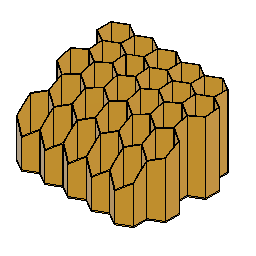
HEXAGON-10 (Autodesk Fusion 360 design; units mm, degrees)
Autodesk Fusion 360 part; units mm, degrees
note: some values were not read from the file. Set by a fixed rule: which sketch regions a step uses.
sketch "Sketch1" plane through (0, 0, 0) normal (0, 1, 0) x (1, 0, 0)
  line L0 (16, 9.2376) -> (0, 18.4752)
  line L1 (0, 18.4752) -> (-16, 9.2376)
  line L2 (-16, -9.2376) -> (0, -18.4752)
  line L3 (0, -18.4752) -> (16, -9.2376)
  line L4 (16, -9.2376) -> (16, 9.2376)
  line L5 (32, -18.4752) -> (48, -9.2376)
  line L6 (48, 9.2376) -> (32, 18.4752)
  line L7 (16, 9.2376) -> (16, -9.2376)
  line L8 (48, -9.2376) -> (48, 9.2376)
  line L9 (32, 18.4752) -> (16, 9.2376)
  line L10 (16, -9.2376) -> (32, -18.4752)
  line L11 (64, -18.4752) -> (80, -9.2376)
  line L12 (80, 9.2376) -> (64, 18.4752)
  line L13 (48, 9.2376) -> (48, -9.2376)
  line L14 (80, -9.2376) -> (80, 9.2376)
  line L15 (64, 18.4752) -> (48, 9.2376)
  line L16 (48, -9.2376) -> (64, -18.4752)
  line L17 (96, -18.4752) -> (112, -9.2376)
  line L18 (112, 9.2376) -> (96, 18.4752)
  line L19 (80, 9.2376) -> (80, -9.2376)
  line L20 (112, -9.2376) -> (112, 9.2376)
  line L21 (96, 18.4752) -> (80, 9.2376)
  line L22 (80, -9.2376) -> (96, -18.4752)
  line L23 (128, -18.4752) -> (144, -9.2376)
  line L24 (144, 9.2376) -> (128, 18.4752)
  line L25 (112, 9.2376) -> (112, -9.2376)
  line L26 (144, -8.7757) -> (144, 9.2376)
  line L27 (128, 18.4752) -> (112, 9.2376)
  line L28 (112, -9.2376) -> (128, -18.4752)
  line L29 (-16, 9.2376) -> (-16, -9.2376)
  line L30 (16, -9.2376) -> (0, -18.4752)
  line L31 (0, -18.4752) -> (0, -36.9504)
  line L32 (0, -36.9504) -> (16, -46.188)
  line L33 (16, -46.188) -> (32, -36.9504)
  line L34 (32, -36.9504) -> (32, -18.4752)
  line L35 (32, -18.4752) -> (16, -9.2376)
  line L36 (32, -18.4752) -> (32, -36.9504)
  line L37 (32, -36.9504) -> (48, -46.188)
  line L38 (48, -46.188) -> (64, -36.9504)
  line L39 (64, -36.9504) -> (64, -18.4752)
  line L40 (64, -18.4752) -> (48, -9.2376)
  line L41 (48, -9.2376) -> (32, -18.4752)
  line L42 (64, -18.4752) -> (64, -36.9504)
  line L43 (64, -36.9504) -> (80, -46.188)
  line L44 (80, -46.188) -> (96, -36.9504)
  line L45 (96, -36.9504) -> (96, -18.4752)
  line L46 (96, -18.4752) -> (80, -9.2376)
  line L47 (80, -9.2376) -> (64, -18.4752)
  line L48 (112, -9.2376) -> (96, -18.4752)
  line L49 (96, -18.4752) -> (96, -36.9504)
  line L50 (96, -36.9504) -> (112, -46.188)
  line L51 (112, -46.188) -> (128, -36.9504)
  line L52 (128, -36.9504) -> (128, -18.4752)
  line L53 (128, -18.4752) -> (112, -9.2376)
  line L54 (128, -18.4752) -> (128, -36.9504)
  line L55 (128, -36.9504) -> (144, -46.188)
  line L56 (144, -46.188) -> (160, -36.9504)
  line L57 (160, -36.9504) -> (160, -18.4752)
  line L58 (160, -18.4752) -> (144, -9.2376)
  line L59 (144, -9.2376) -> (128, -18.4752)
  line L60 (0, -36.9504) -> (-16, -46.188)
  line L61 (-16, -46.188) -> (-16, -64.6632)
  line L62 (-16, -64.6632) -> (0, -73.9008)
  line L63 (0, -73.9008) -> (16, -64.6632)
  line L64 (16, -64.6632) -> (16, -46.188)
  line L65 (16, -46.188) -> (0, -36.9504)
  line L66 (16, -46.188) -> (16, -64.6632)
  line L67 (16, -64.6632) -> (32, -73.9008)
  line L68 (32, -73.9008) -> (48, -64.6632)
  line L69 (48, -64.6632) -> (48, -46.188)
  line L70 (48, -46.188) -> (32, -36.9504)
  line L71 (32, -36.9504) -> (16, -46.188)
  line L72 (48, -64.6632) -> (64, -73.9008)
  line L73 (64, -73.9008) -> (80, -64.6632)
  line L74 (80, -64.6632) -> (80, -46.188)
  line L75 (80, -46.188) -> (64, -36.9504)
  line L76 (64, -36.9504) -> (48, -46.188)
  line L77 (48, -46.188) -> (48, -64.6632)
  line L78 (80, -64.6632) -> (96, -73.9008)
  line L79 (96, -73.9008) -> (112, -64.6632)
  line L80 (112, -64.6632) -> (112, -46.188)
  line L81 (112, -46.188) -> (96, -36.9504)
  line L82 (96, -36.9504) -> (80, -46.188)
  line L83 (80, -46.188) -> (80, -64.6632)
  line L84 (112, -64.6632) -> (128, -73.9008)
  line L85 (128, -73.9008) -> (144, -64.6632)
  line L86 (144, -64.6632) -> (144, -46.188)
  line L87 (144, -46.188) -> (128, -36.9504)
  line L88 (128, -36.9504) -> (112, -46.188)
  line L89 (112, -46.188) -> (112, -64.6632)
  line L90 (0, -73.9008) -> (0, -92.376)
  line L91 (0, -92.376) -> (16, -101.6136)
  line L92 (16, -101.6136) -> (32, -92.376)
  line L93 (32, -92.376) -> (32, -73.9008)
  line L94 (32, -73.9008) -> (16, -64.6632)
  line L95 (16, -64.6632) -> (0, -73.9008)
  line L96 (32, -73.9008) -> (32, -92.376)
  line L97 (32, -92.376) -> (48, -101.6136)
  line L98 (48, -101.6136) -> (64, -92.376)
  line L99 (64, -92.376) -> (64, -73.9008)
  line L100 (64, -73.9008) -> (48, -64.6632)
  line L101 (48, -64.6632) -> (32, -73.9008)
  line L102 (64, -92.376) -> (80, -101.6136)
  line L103 (80, -101.6136) -> (96, -92.376)
  line L104 (96, -92.376) -> (96, -73.9008)
  line L105 (96, -73.9008) -> (80, -64.6632)
  line L106 (80, -64.6632) -> (64, -73.9008)
  line L107 (64, -73.9008) -> (64, -92.376)
  line L108 (96, -92.376) -> (112, -101.6136)
  line L109 (112, -101.6136) -> (128, -92.376)
  line L110 (128, -92.376) -> (128, -73.9008)
  line L111 (128, -73.9008) -> (112, -64.6632)
  line L112 (112, -64.6632) -> (96, -73.9008)
  line L113 (96, -73.9008) -> (96, -92.376)
  line L114 (128, -92.376) -> (128, -73.9008)
  line L115 (128, -73.9008) -> (112, -64.6632)
  line L116 (112, -64.6632) -> (96, -73.9008)
  line L117 (96, -73.9008) -> (96, -92.376)
  line L118 (96, -92.376) -> (112, -101.6136)
  line L119 (112, -101.6136) -> (128, -92.376)
  line L120 (16, -101.6136) -> (0, -92.376)
  line L121 (0, -92.376) -> (-16, -101.6136)
  line L122 (-16, -101.6136) -> (-16, -120.0889)
  line L123 (-16, -120.0889) -> (0, -129.3265)
  line L124 (0, -129.3265) -> (16, -120.0889)
  line L125 (16, -120.0889) -> (16, -101.6136)
  line L126 (16, -101.6136) -> (16, -120.0889)
  line L127 (16, -120.0889) -> (32, -129.3265)
  line L128 (32, -129.3265) -> (48, -120.0889)
  line L129 (48, -120.0889) -> (48, -101.6136)
  line L130 (48, -101.6136) -> (32, -92.376)
  line L131 (32, -92.376) -> (16, -101.6136)
  line L132 (48, -120.0889) -> (64, -129.3265)
  line L133 (64, -129.3265) -> (80, -120.0889)
  line L134 (80, -120.0889) -> (80, -101.6136)
  line L135 (80, -101.6136) -> (64, -92.376)
  line L136 (64, -92.376) -> (48, -101.6136)
  line L137 (48, -101.6136) -> (48, -120.0889)
  line L138 (80, -101.6136) -> (80, -120.0889)
  line L139 (80, -120.0889) -> (96, -129.3265)
  line L140 (96, -129.3265) -> (112, -120.0889)
  line L141 (112, -120.0889) -> (112, -101.6136)
  line L142 (112, -101.6136) -> (96, -92.376)
  line L143 (96, -92.376) -> (80, -101.6136)
  line L144 (112, -101.6136) -> (112, -120.0889)
  line L145 (112, -120.0889) -> (128, -129.3265)
  line L146 (128, -129.3265) -> (144, -120.0889)
  line L147 (144, -120.0889) -> (144, -101.6136)
  line L148 (144, -101.6136) -> (128, -92.376)
  line L149 (128, -92.376) -> (112, -101.6136)
  line L150 (144, -64.6632) -> (128, -73.9008)
  line L151 (128, -73.9008) -> (128, -92.376)
  line L152 (128, -92.376) -> (144, -101.6136)
  line L153 (144, -101.6136) -> (160, -92.376)
  line L154 (160, -92.376) -> (160, -73.9008)
  line L155 (160, -73.9008) -> (144, -64.6632)
  line L156 (-16.8, 9.6995) -> (-16.8, -9.6995)
  line L157 (-16.8, -9.6995) -> (-0.8, -18.9371)
  line L158 (-0.8, -18.9371) -> (-0.8, -36.4885)
  line L159 (-0.8, -36.4885) -> (-16.8, -45.7261)
  line L160 (-16.8, -45.7261) -> (-16.8, -65.1251)
  line L161 (-16.8, -65.1251) -> (-0.8, -74.3627)
  line L162 (-0.8, -74.3627) -> (-0.8, -91.9142)
  line L163 (-0.8, -91.9142) -> (-16.8, -101.1518)
  line L164 (-16.8, -101.1518) -> (-16.8, -120.5507)
  line L165 (-16.8, -120.5507) -> (0, -130.2502)
  line L166 (0, -130.2502) -> (16, -121.0126)
  line L167 (16, -121.0126) -> (32, -130.2502)
  line L168 (32, -130.2502) -> (48, -121.0126)
  line L169 (48, -121.0126) -> (64, -130.2502)
  line L170 (64, -130.2502) -> (80, -121.0126)
  line L171 (80, -121.0126) -> (96, -130.2502)
  line L172 (96, -130.2502) -> (112, -121.0126)
  line L173 (112, -121.0126) -> (128, -130.2502)
  line L174 (128, -130.2502) -> (144.8, -120.5507)
  line L175 (144.8, -120.5507) -> (144.8, -102.0755)
  line L176 (144.8, -102.0755) -> (160.8, -92.8379)
  line L177 (160.8, -92.8379) -> (160.8, -73.439)
  line L178 (160.8, -73.439) -> (144.8, -64.2013)
  line L179 (144.8, -64.2013) -> (144.8, -46.6499)
  line L180 (144.8, -46.6499) -> (160.8, -37.4123)
  line L181 (160.8, -37.4123) -> (160.8, -18.0133)
  line L182 (160.8, -18.0133) -> (144.8, -8.7757)
  line L183 (144.8, -8.7757) -> (144.8, 9.6995)
  line L184 (144.8, 9.6995) -> (128, 19.399)
  line L185 (128, 19.399) -> (112, 10.1614)
  line L186 (112, 10.1614) -> (96, 19.399)
  line L187 (96, 19.399) -> (80, 10.1614)
  line L188 (80, 10.1614) -> (64, 19.399)
  line L189 (64, 19.399) -> (48, 10.1614)
  line L190 (48, 10.1614) -> (32, 19.399)
  line L191 (32, 19.399) -> (16, 10.1614)
  line L192 (16, 10.1614) -> (0, 19.399)
  line L193 (0, 19.399) -> (-16.8, 9.6995)
  line L194 (15.6, -9.0067) -> (15.6, 9.4685)
  line L195 (15.6, -9.0067) -> (-0.4, -18.2443)
  line L196 (32.4, -18.2443) -> (16.4, -9.0067)
  line L197 (16.4, -9.0067) -> (16.4, 9.4685)
  line L198 (48.4, -9.0067) -> (48.4, 9.4685)
  line L199 (48.4, -9.0067) -> (64.2, -18.1288)
  line L200 (47.6, -9.4685) -> (47.6, 9.4685)
  line L201 (63.8, -18.1288) -> (79.6, -9.0067)
  line L202 (79.6, -9.0067) -> (79.6, 9.4685)
  line L203 (96.2, -18.1288) -> (80.4, -9.0067)
  line L204 (80.4, -9.0067) -> (80.4, 9.4685)
  line L205 (111.6, 9.4685) -> (111.6, -9.0067)
  line L206 (111.6, -9.0067) -> (95.8, -18.1288)
  line L207 (112.4, 9.4685) -> (112.4, -9.0067)
  line L208 (112.4, -9.0067) -> (128, -18.0133)
  line L209 (144, -8.7757) -> (128, -18.0133)
  line L210 (32.4, -18.7061) -> (32.4, -36.7195)
  line L211 (32.4, -36.7195) -> (48, -45.7261)
  line L212 (48, -45.7261) -> (63.6, -36.7195)
  line L213 (63.6, -36.7195) -> (63.6, -18.7061)
  line L214 (63.6, -18.7061) -> (48, -9.6995)
  line L215 (48, -9.6995) -> (32.4, -18.7061)
  line L216 (16, -45.7261) -> (0, -36.4885)
  line L217 (16, -45.7261) -> (31.6, -36.7195)
  line L218 (31.6, -18.7061) -> (31.6, -36.7195)
  line L219 (31.6, -18.7061) -> (16, -9.6995)
  line L220 (16, -9.6995) -> (0, -18.9371)
  line L221 (80, -9.6995) -> (64.4, -18.7061)
  line L222 (64.4, -36.7195) -> (64.4, -18.7061)
  line L223 (64.4, -36.7195) -> (80, -45.7261)
  line L224 (95.6, -36.7195) -> (80, -45.7261)
  line L225 (95.6, -18.7061) -> (95.6, -36.7195)
  line L226 (95.6, -18.7061) -> (80, -9.6995)
  line L227 (96.4, -36.7195) -> (96.4, -18.7061)
  line L228 (112, -9.6995) -> (96.4, -18.7061)
  line L229 (112, -9.6995) -> (127.6, -18.7061)
  line L230 (127.6, -36.7195) -> (127.6, -18.7061)
  line L231 (112, -45.7261) -> (127.6, -36.7195)
  line L232 (112, -45.7261) -> (96.4, -36.7195)
  line L233 (144.4, -9.4685) -> (128.4, -18.7061)
  line L234 (128.4, -36.7195) -> (128.4, -18.7061)
  line L235 (128.4, -36.7195) -> (144.4, -45.9571)
  line L236 (15.6, -46.419) -> (15.6, -64.4323)
  line L237 (15.6, -64.4323) -> (-0.4, -73.6699)
  line L238 (32, -73.439) -> (47.6, -64.4323)
  line L239 (47.6, -64.4323) -> (47.6, -46.419)
  line L240 (47.6, -46.419) -> (32, -37.4123)
  line L241 (16.4, -46.419) -> (32, -37.4123)
  line L242 (16.4, -46.419) -> (16.4, -64.4323)
  line L243 (32, -73.439) -> (16.4, -64.4323)
  line L244 (48.4, -64.4323) -> (48.4, -46.419)
  line L245 (64, -37.4123) -> (48.4, -46.419)
  line L246 (64, -37.4123) -> (79.6, -46.419)
  line L247 (79.6, -64.4323) -> (79.6, -46.419)
  line L248 (64, -73.439) -> (79.6, -64.4323)
  line L249 (64, -73.439) -> (48.4, -64.4323)
  line L250 (111.6, -46.419) -> (96, -37.4123)
  line L251 (80.4, -46.419) -> (96, -37.4123)
  line L252 (80.4, -46.419) -> (80.4, -64.4323)
  line L253 (80.4, -64.4323) -> (96, -73.439)
  line L254 (96, -73.439) -> (111.6, -64.4323)
  line L255 (111.6, -64.4323) -> (111.6, -46.419)
  line L256 (144, -46.6499) -> (128, -37.4123)
  line L257 (112.4, -46.419) -> (128, -37.4123)
  line L258 (112.4, -64.4323) -> (112.4, -46.419)
  line L259 (128, -73.439) -> (112.4, -64.4323)
  line L260 (144, -64.2013) -> (128, -73.439)
  line L261 (0, -91.9142) -> (16, -101.1518)
  line L262 (31.6, -92.1451) -> (16, -101.1518)
  line L263 (31.6, -92.1451) -> (31.6, -74.1318)
  line L264 (16, -65.1251) -> (31.6, -74.1318)
  line L265 (0, -74.3627) -> (16, -65.1251)
  line L266 (48, -65.1251) -> (32.4, -74.1318)
  line L267 (32.4, -74.1318) -> (32.4, -92.1451)
  line L268 (48, -101.1518) -> (32.4, -92.1451)
  line L269 (63.6, -92.1451) -> (48, -101.1518)
  line L270 (63.6, -74.1318) -> (63.6, -92.1451)
  line L271 (63.6, -74.1318) -> (48, -65.1251)
  line L272 (80, -65.1251) -> (95.6, -74.1318)
  line L273 (95.6, -74.1318) -> (95.6, -92.1451)
  line L274 (95.6, -92.1451) -> (80, -101.1518)
  line L275 (64.4, -92.1451) -> (80, -101.1518)
  line L276 (64.4, -74.1318) -> (64.4, -92.1451)
  line L277 (80, -65.1251) -> (64.4, -74.1318)
  line L278 (112, -65.1251) -> (96.4, -74.1318)
  line L279 (96.4, -92.1451) -> (96.4, -74.1318)
  line L280 (96.4, -92.1451) -> (112, -101.1518)
  line L281 (127.6, -92.1451) -> (112, -101.1518)
  line L282 (127.6, -92.1451) -> (127.6, -74.1318)
  line L283 (112, -65.1251) -> (127.6, -74.1318)
  line L284 (144.4, -64.8942) -> (128.4, -74.1318)
  line L285 (128.4, -92.1451) -> (128.4, -74.1318)
  line L286 (128.4, -92.1451) -> (144.4, -101.3827)
  line L287 (-0.4, -92.607) -> (15.6, -101.8446)
  line L288 (15.6, -101.8446) -> (15.6, -120.3198)
  line L289 (47.6, -120.3198) -> (47.6, -101.8446)
  line L290 (47.6, -101.8446) -> (32, -92.8379)
  line L291 (16.4, -101.8446) -> (32, -92.8379)
  line L292 (16.4, -101.8446) -> (16.4, -120.3198)
  line L293 (79.6, -120.3198) -> (79.6, -101.8446)
  line L294 (64, -92.8379) -> (79.6, -101.8446)
  line L295 (64, -92.8379) -> (48.4, -101.8446)
  line L296 (48.4, -101.8446) -> (48.4, -120.3198)
  line L297 (80.4, -120.3198) -> (80.4, -101.8446)
  line L298 (80.4, -101.8446) -> (96, -92.8379)
  line L299 (96, -92.8379) -> (111.6, -101.8446)
  line L300 (111.6, -101.8446) -> (111.6, -120.3198)
  line L301 (112.4, -120.3198) -> (112.4, -101.8446)
  line L302 (112.4, -101.8446) -> (128, -92.8379)
  line L303 (128, -92.8379) -> (144, -102.0755)
  line L304 (-0.4, -37.1814) -> (15.6, -46.419)
  point P0 (32, 0)
  point P1 (32, 0)
  point P2 (64, 0)
  point P3 (64, 0)
  point P4 (96, 0)
  point P5 (96, 0)
  point P6 (128, 0)
  point P7 (128, 0)
  point P8 (16, -27.7128)
  point P9 (48, -27.7128)
  point P10 (80, -27.7128)
  point P11 (112, -27.7128)
  point P12 (144, -27.7128)
  point P13 (0, -55.4256)
  point P14 (32, -55.4256)
  point P15 (64, -55.4256)
  point P16 (96, -55.4256)
  point P17 (128, -55.4256)
  point P18 (16, -83.1384)
  point P19 (48, -83.1384)
  point P20 (80, -83.1384)
  point P21 (112, -83.1384)
  point P22 (112, -83.1384)
  point P23 (0, -110.8513)
  point P24 (32, -110.8513)
  point P25 (64, -110.8513)
  point P26 (96, -110.8513)
  point P27 (128, -110.8513)
  point P28 (144, -83.1384)
  dimension "d10" = 16
  dimension "d28" = 0.8
  dimension "d38" = -0.4
  dimension "d40" = -0.4
  dimension "d41" = 0.4
  dimension "d44" = -0.4
  dimension "d45" = 0.4
  dimension "d46" = -0.4
  dimension "d49" = -0.4
  dimension "d50" = 0.4
  dimension "d51" = -0.4
  constraint parallel L59 L209
  constraint parallel L25 L207
  constraint parallel L28 L208
  constraint parallel L25 L205
  constraint parallel L48 L206
  constraint coincident L18 L205.start
  constraint parallel L46 L203
  constraint parallel L14 L204
  constraint parallel L11 L201
  constraint parallel L14 L202
  constraint coincident L12 L202.end
  constraint parallel L4 L194
  constraint parallel L30 L195
  constraint coincident L0 L194.end
  constraint parallel L35 L196
  constraint parallel L4 L197
  constraint coincident L9 L197.end
  constraint parallel L8 L198
  constraint parallel L16 L199
  constraint parallel L8 L200
  constraint coincident L6 L200.end
  constraint parallel L150 L284
  constraint parallel L110 L285
  constraint parallel L152 L286
  constraint parallel L141 L301
  constraint parallel L119 L302
  constraint parallel L152 L303
  constraint parallel L134 L297
  constraint parallel L103 L298
  constraint parallel L108 L299
  constraint parallel L144 L300
  constraint coincident L140 L300.end
  constraint parallel L134 L293
  constraint parallel L102 L294
  constraint parallel L136 L295
  constraint parallel L137 L296
  constraint parallel L129 L289
  constraint parallel L130 L290
  constraint parallel L92 L291
  constraint parallel L126 L292
  constraint parallel L91 L287
  constraint parallel L126 L288
  constraint coincident L127 L292.end
  constraint parallel L91 L261
  constraint parallel L131 L262
  constraint parallel L93 L263
  constraint parallel L67 L264
  constraint parallel L63 L265
  constraint parallel L65 L216
  constraint parallel L33 L217
  constraint parallel L36 L218
  constraint parallel L35 L219
  constraint parallel L30 L220
  constraint coincident L31 L216.end
  constraint parallel L66 L236
  constraint parallel L95 L237
  constraint coincident L62 L237.end
  constraint parallel L59 L233
  constraint parallel L52 L234
  constraint parallel L55 L235
  constraint coincident L56 L235.end
  constraint parallel L87 L256
  constraint parallel L51 L257
  constraint parallel L80 L258
  constraint parallel L115 L259
  constraint parallel L150 L260
  constraint coincident L5 L200.start
  constraint parallel L32 L304
  constraint coincident L2 L195.end
  constraint coincident L31 L220.end
  constraint coincident L5 L196.start
  measures "d10" distance of origin L4
extrude "Extrude1" add sketch "Sketch1" along normal blind 100 contours L0 L2 L3 L4 L7 L30 L194 L195 | L4 L5 L7 L9 L10 L35 L41 L196 L197 | L3 L10 L30 L31 L32 L33 L34 L35 L36 L65 L71 L216 L217 L218 L219 L220 | L5 L16 L34 L36 L37 L38 L39 L40 L41 L42 L70 L76 | L33 L37 L64 L66 L67 L68 L69 L70 L71 L77 L94 L101 | L5 L6 L8 L13 L41 L200 | L32 L60 L62 L63 L64 L65 L66 L95 L236 L237 L304 | L38 L43 L69 L72 L73 L74 L75 L76 L77 L83 L100 L106 | L8 L11 L12 L13 L14 L15 L16 L19 L40 L47 L198 L199 L201 L202 | L63 L67 L90 L91 L92 L93 L94 L95 L96 L120 L131 L261 L262 L263 L264 L265 | L11 L22 L39 L42 L43 L44 L45 L46 L47 L49 L75 L82 | L68 L72 L93 L96 L97 L98 L99 L100 L101 L107 L130 L136 | L44 L50 L74 L78 L79 L80 L81 L82 L83 L89 L105 L112 L116 | L73 L78 L99 L102 L103 L104 L105 L106 L107 L113 L117 L135 L143 | L14 L17 L18 L19 L20 L21 L22 L25 L46 L48 L203 L204 L205 L206 | L92 L97 L125 L126 L127 L128 L129 L130 L131 L137 L289 L290 L291 L292 | L17 L28 L45 L48 L49 L50 L51 L52 L53 L54 L81 L88 | L98 L102 L129 L132 L133 L134 L135 L136 L137 L138 L293 L294 L295 L296 | L91 L120 L121 L124 L125 L126 L287 L288 | L51 L55 L80 L84 L85 L86 L87 L88 L89 L111 L115 L150 L256 L257 L258 L259 L260 | L79 L84 L104 L108 L109 L110 L111 L112 L113 L114 L115 L116 L117 L118 L119 L142 L149 L151 | L103 L108 L118 L134 L138 L139 L140 L141 L142 L143 L144 L297 L298 L299 L300 | L23 L52 L54 L55 L56 L58 L59 L87 L233 L234 L235 | L85 L110 L114 L148 L150 L151 L152 L153 L155 L284 L285 L286 | L109 L119 L141 L144 L145 L147 L148 L149 L152 L301 L302 L303 | L156 L157 L158 L159 L160 L161 L162 L163 L164 L165 L166 L167 L168 L169 L170 L171 L172 L173 L174 L175 L176 L177 L178 L179 L180 L181 L182 L183 L184 L185 L186 L187 L188 L189 L190 L191 L192 L193 makes body 1
extrude "Extrude2" add sketch "Sketch1" along normal blind 1.6 separate body contours L0 L2 L3 L4 L7 L30 L194 L195 | L4 L5 L7 L9 L10 L35 L41 L196 L197 | L0 L1 L2 L29 L194 L195 | L3 L10 L30 L31 L32 L33 L34 L35 L36 L65 L71 L216 L217 L218 L219 L220 | L5 L6 L9 L41 L196 L197 L200 | L5 L16 L34 L36 L37 L38 L39 L40 L41 L42 L70 L76 | L31 L216 L217 L218 L219 L220 | L33 L37 L64 L66 L67 L68 L69 L70 L71 L77 L94 L101 | L5 L6 L8 L13 L41 L200 | L32 L60 L62 L63 L64 L65 L66 L95 L236 L237 L304 | L38 L43 L69 L72 L73 L74 L75 L76 L77 L83 L100 L106 | L8 L11 L12 L13 L14 L15 L16 L19 L40 L47 L198 L199 L201 L202 | L63 L67 L90 L91 L92 L93 L94 L95 L96 L120 L131 L261 L262 L263 L264 L265 | L11 L22 L39 L42 L43 L44 L45 L46 L47 L49 L75 L82 | L68 L72 L93 L96 L97 L98 L99 L100 L101 L107 L130 L136 | L12 L15 L198 L199 L201 L202 | L60 L61 L62 L236 L237 L304 | L44 L50 L74 L78 L79 L80 L81 L82 L83 L89 L105 L112 L116 | L73 L78 L99 L102 L103 L104 L105 L106 L107 L113 L117 L135 L143 | L14 L17 L18 L19 L20 L21 L22 L25 L46 L48 L203 L204 L205 L206 | L90 L261 L262 L263 L264 L265 | L92 L97 L125 L126 L127 L128 L129 L130 L131 L137 L289 L290 L291 L292 | L17 L28 L45 L48 L49 L50 L51 L52 L53 L54 L81 L88 | L98 L102 L129 L132 L133 L134 L135 L136 L137 L138 L293 L294 L295 L296 | L91 L120 L121 L124 L125 L126 L287 L288 | L51 L55 L80 L84 L85 L86 L87 L88 L89 L111 L115 L150 L256 L257 L258 L259 L260 | L79 L84 L104 L108 L109 L110 L111 L112 L113 L114 L115 L116 L117 L118 L119 L142 L149 L151 | L103 L108 L118 L134 L138 L139 L140 L141 L142 L143 L144 L297 L298 L299 L300 | L18 L21 L203 L204 L205 L206 | L23 L52 L54 L55 L56 L58 L59 L87 L233 L234 L235 | L121 L122 L123 L124 L287 L288 | L127 L128 L289 L290 L291 L292 | L132 L133 L293 L294 L295 L296 | L85 L110 L114 L148 L150 L151 L152 L153 L155 L284 L285 L286 | L109 L119 L141 L144 L145 L147 L148 L149 L152 L301 L302 L303 | L139 L140 L297 L298 L299 L300 | L56 L57 L58 L233 L234 L235 | L86 L256 L257 L258 L259 L260 | L153 L154 L155 L284 L285 L286 | L145 L146 L147 L301 L302 L303 | L24 L26 L27 L207 L208 L209 | L156 L157 L158 L159 L160 L161 L162 L163 L164 L165 L166 L167 L168 L169 L170 L171 L172 L173 L174 L175 L176 L177 L178 L179 L180 L181 L182 L183 L184 L185 L186 L187 L188 L189 L190 L191 L192 L193 | L210 L211 L212 L213 L214 L215 | L221 L222 L223 L224 L225 L226 | L227 L228 L229 L230 L231 L232 | L238 L239 L240 L241 L242 L243 | L244 L245 L246 L247 L248 L249 | L250 L251 L252 L253 L254 L255 | L266 L267 L268 L269 L270 L271 | L272 L273 L274 L275 L276 L277 | L278 L279 L280 L281 L282 L283 makes body 2
sketch "Sketch2" plane through (0, 0, 0) normal (1, 0, 0) x (0, 0, -1)
  line L0 (9.6995, 0) -> (19.399, 0) construction
  line L1 (19.399, 0) -> (19.399, 100) construction
  line L2 (19.399, 100) -> (9.6995, 100) construction
  line L3 (9.6995, 100) -> (9.6995, 0) construction
  line L4 (-130.2502, 0) -> (-120.5507, 0) construction
  line L5 (-120.5507, 0) -> (-120.5507, 100) construction
  line L6 (-120.5507, 100) -> (-130.2502, 100) construction
  line L7 (-130.2502, 100) -> (-130.2502, 0) construction
  line L8 (19.399, 100) -> (19.399, 0)
  line L9 (19.399, 0) -> (-130.2502, 0)
  line L10 (-130.2502, 0) -> (-130.2502, 40)
  line L11 (19.399, 100) -> (-130.2502, 100)
  line L12 (-130.2502, 100) -> (-130.2502, 40)
  arc A0 (-15.359, 100) -> (-130.2502, 40) centre (-15.359, -40) ccw
  dimension "d71" = 40
  dimension "d73" = 140
  dimension "d74" = 34.7579
  constraint coincident L1.end L2.start
  constraint coincident L0.end L1.start
  constraint coincident L4.start L7.end
  constraint coincident L7 L10.end
  constraint perpendicular L4 L10
  constraint coincident L6.end L7.start
  constraint tangent L11 A0
  constraint coincident L11 A0.start
  measures "d71" distance of L4.start L10.end
  measures "d73" radius of A0
  measures "d74" distance of L1.end A0.start
extrude "Extrude4" cut sketch "Sketch2" along normal blind 193 and the other way blind 65 contours L11 L12 A0 bodies 1
copy_body "Body->Comp1" bodies 1 removing the originals makes body 3 in component "Component"
copy_body "Body->Comp2" bodies 2 removing the originals makes body 4 in component "Component'"
component "Component" placed x (1, 0, 0) y (0, 1, 0) z (0, 0, 1) at (0, 0, 0)
component "Component'" placed x (1, 0, 0) y (0, 1, 0) z (0, 0, 1) at (0, 0, 0)
